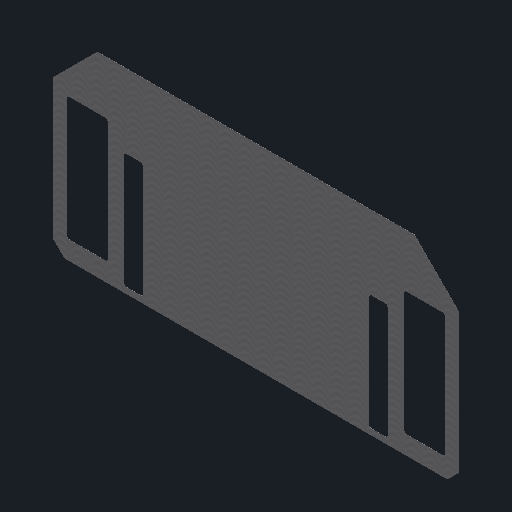
# Autodesk Inventor part: PlanchaBaseInferior
Saved by Autodesk Inventor 2022 (Build 260153000, 153)
## iProperties
Created: 2021-09-22
Part Number: PlanchaBaseInferior
Material: Steel, Mild, Welded
Document SubType Name: Sheet Metal
Designer: Andres
Density: 7.85 g/cm^3
Sheet Metal Rule: Default_mm
Appearance: Weld - Steel Mild
Author: Andres
Autodesk Inventor part; units mm, degrees
ref_plane "YZ Plane" through (0, 0, 0) normal (1, 0, 0) x (0, 1, 0)
ref_plane "XZ Plane" through (0, 0, 0) normal (0, 1, 0) x (-1, 0, 0)
ref_plane "XY Plane" through (0, 0, 0) normal (0, 0, 1) x (1, 0, 0)
sketch "Sketch1" plane through (0, 0, 0) normal (0, 0, 1) x (1, 0, 0)
  line L0 (893.3076, -345.9853) -> (750.9853, -345.9853)
  line L1 (-16.337, -345.9853) -> (-29.0147, -333.3076)
  line L2 (-29.0147, -333.3076) -> (-29.0147, -13.663)
  line L3 (-29.0147, -13.663) -> (63.663, 79.0147)
  line L4 (63.663, 79.0147) -> (125.9853, 79.0147)
  line L5 (750.9853, 79.0147) -> (813.3076, 79.0147)
  line L6 (570.9853, 79.0147) -> (725.9853, 79.0147)
  line L7 (150.9853, 79.0147) -> (305.9853, 79.0147)
  line L8 (330.9853, 79.0147) -> (545.9853, 79.0147)
  line L9 (813.3076, 79.0147) -> (905.9853, -13.663)
  line L10 (905.9853, -13.663) -> (905.9853, -333.3076)
  line L11 (905.9853, -333.3076) -> (893.3076, -345.9853)
  line L12 (125.9853, -345.9853) -> (-16.337, -345.9853)
  line L13 (903.663, -370.9853) -> (750.9853, -370.9853)
  line L14 (930.9853, -343.663) -> (903.663, -370.9853)
  line L15 (930.9853, -3.3076) -> (930.9853, -343.663)
  line L16 (823.663, 104.0147) -> (930.9853, -3.3076)
  line L17 (53.3076, 104.0147) -> (823.663, 104.0147)
  line L18 (-54.0147, -3.3076) -> (53.3076, 104.0147)
  line L19 (-54.0147, -343.663) -> (-54.0147, -3.3076)
  line L20 (-26.6924, -370.9853) -> (-54.0147, -343.663)
  line L21 (125.9853, -370.9853) -> (-26.6924, -370.9853)
  line L22 (750.9853, -370.9853) -> (125.9853, -370.9853)
  line L23 (125.9853, -370.9853) -> (125.9853, -345.9853)
  line L24 (125.9853, 79.0147) -> (125.9853, 91.5147)
  line L25 (125.9853, 91.5147) -> (150.9853, 91.5147)
  line L26 (150.9853, 79.0147) -> (150.9853, 91.5147)
  line L27 (305.9853, 91.5147) -> (305.9853, 79.0147)
  line L28 (305.9853, 91.5147) -> (330.9853, 91.5147)
  line L29 (330.9853, 91.5147) -> (330.9853, 79.0147)
  line L30 (545.9853, 91.5147) -> (545.9853, 79.0147)
  line L31 (545.9853, 91.5147) -> (570.9853, 91.5147)
  line L32 (570.9853, 91.5147) -> (570.9853, 79.0147)
  line L33 (725.9853, 79.0147) -> (725.9853, 91.5147)
  line L34 (725.9853, 91.5147) -> (750.9853, 91.5147)
  line L35 (750.9853, 79.0147) -> (750.9853, 91.5147)
  line L36 (750.9853, -370.9853) -> (750.9853, -345.9853)
extrude "Plate1" add sketch "Sketch1" along normal blind 0.5
sketch "Sketch2" plane through (0, 0, 0.5) normal (0, 0, 1) x (1, 0, 0)
  line L0 (78.4853, -25.4853) -> (-21.5147, -25.4853)
  line L1 (-21.5147, -25.4853) -> (-21.5147, -325.4853)
  line L2 (-21.5147, -325.4853) -> (78.4853, -325.4853)
  line L3 (78.4853, -325.4853) -> (78.4853, -25.4853)
  line L4 (78.4853, -25.4853) -> (-21.5147, -325.4853) construction
  line L5 (-21.5147, -25.4853) -> (78.4853, -325.4853) construction
  line L6 (119.5571, -370.4853) -> (-26.4853, -370.4853)
  line L7 (-26.4853, -370.4853) -> (-53.5147, -343.4558)
  line L8 (-53.5147, -343.4558) -> (-53.5147, -3.5147)
  line L9 (-53.5147, -3.5147) -> (53.5147, 103.5147)
  line L10 (53.5147, 103.5147) -> (823.4558, 103.5147)
  line L11 (823.4558, 103.5147) -> (930.4853, -3.5147)
  line L12 (930.4853, -3.5147) -> (930.4853, -343.4558)
  line L13 (930.4853, -343.4558) -> (903.4558, -370.4853)
  line L14 (903.4558, -370.4853) -> (757.4135, -370.4853)
  line L15 (893.5147, -346.4853) -> (757.4135, -346.4853)
  line L16 (906.4853, -333.5147) -> (893.5147, -346.4853)
  line L17 (906.4853, -13.4558) -> (906.4853, -333.5147)
  line L18 (813.5147, 79.5147) -> (906.4853, -13.4558)
  line L19 (757.4135, 79.5147) -> (813.5147, 79.5147)
  line L20 (577.4135, 79.5147) -> (719.5571, 79.5147)
  line L21 (337.4135, 79.5147) -> (539.5571, 79.5147)
  line L22 (63.4558, 79.5147) -> (119.5571, 79.5147)
  line L23 (157.4135, 79.5147) -> (299.5571, 79.5147)
  line L24 (-29.5147, -13.4558) -> (63.4558, 79.5147)
  line L25 (-29.5147, -333.5147) -> (-29.5147, -13.4558)
  line L26 (-16.5442, -346.4853) -> (-29.5147, -333.5147)
  line L27 (119.5571, -346.4853) -> (-16.5442, -346.4853)
  line L28 (438.4853, 188.8971) -> (438.4853, -449.5258) construction
  line L29 (798.4853, -25.4853) -> (898.4853, -25.4853)
  line L30 (898.4853, -25.4853) -> (898.4853, -325.4853)
  line L31 (898.4853, -325.4853) -> (798.4853, -325.4853)
  line L32 (798.4853, -325.4853) -> (798.4853, -25.4853)
  line L33 (798.4853, -25.4853) -> (898.4853, -325.4853) construction
  line L34 (898.4853, -25.4853) -> (798.4853, -325.4853) construction
  line L35 (119.5571, -346.4853) -> (119.5571, -370.4853)
  line L36 (757.4135, -370.4853) -> (757.4135, -346.4853)
  line L37 (757.4135, 79.5147) -> (757.4135, 91.5147)
  line L38 (757.4135, 91.5147) -> (719.5571, 91.5147)
  line L39 (719.5571, 91.5147) -> (719.5571, 79.5147)
  line L40 (577.4135, 79.5147) -> (577.4135, 91.5147)
  line L41 (577.4135, 91.5147) -> (539.5571, 91.5147)
  line L42 (539.5571, 91.5147) -> (539.5571, 79.5147)
  line L43 (337.4135, 79.5147) -> (337.4135, 91.5147)
  line L44 (337.4135, 91.5147) -> (299.5571, 91.5147)
  line L45 (299.5571, 91.5147) -> (299.5571, 79.5147)
  line L46 (157.4135, 79.5147) -> (157.4135, 91.5147)
  line L47 (157.4135, 91.5147) -> (119.5571, 91.5147)
  line L48 (119.5571, 91.5147) -> (119.5571, 79.5147)
  point P0 (0, 0)
  point P1 (28.4853, -175.4853)
  point P2 (438.4853, 79.5147)
  point P3 (848.4853, -175.4853)
  dimension "d1" = 100
  dimension "d2" = 300
  dimension "d4" = 410
  dimension "d5" = 255
  constraints: 96 end point, 5 midpoint, 5 symmetric about line, 2 parallel, 1 horizontal, 1 perpendicular, 1 vertical, 1 vertical alignment, 3 other
  measures "d1" distance between parallel lines of L1 L3
  measures "d2" distance between parallel lines of L2 L0
  measures "d4" distance from line of point (28.485, -175.485) L28
  measures "d5" vertical distance of point (438.485, 79.515) point (28.485, -175.485)
extrude "Cut1" cut sketch "Sketch2" against normal through all contours L3 L2 L1 L0 | L29 L30 L31 L32
fillet "Corner Round1" radius 6 8 edges at (78.4853, -25.4853, 0.25) (-21.5147, -25.4853, 0.25) (-21.5147, -325.4853, 0.25) (78.4853, -325.4853, 0.25) (898.4853, -25.4853, 0.25) (798.4853, -25.4853, 0.25) (898.4853, -325.4853, 0.25) (798.4853, -325.4853, 0.25)
sketch "Boceto3" plane through (0, 0, 0.5) normal (0, 0, 1) x (1, 0, 0)
  line L0 (123.4853, -355.9853) -> (158.4853, -355.9853)
  line L1 (163.4853, -350.9853) -> (163.4853, -80.9853)
  line L2 (158.4853, -75.9853) -> (123.4853, -75.9853)
  line L3 (118.4853, -80.9853) -> (118.4853, -350.9853)
  line L4 (78.4853, -31.4853) -> (78.4853, -319.4853) projected
  line L5 (438.4853, 103.5147) -> (438.4853, -370.4853)
  line L6 (753.4853, -355.9853) -> (718.4853, -355.9853)
  line L7 (713.4853, -350.9853) -> (713.4853, -80.9853)
  line L8 (718.4853, -75.9853) -> (753.4853, -75.9853)
  line L9 (758.4853, -80.9853) -> (758.4853, -350.9853)
  arc A0 (158.4853, -355.9853) -> (163.4853, -350.9853) centre (158.4853, -350.9853) ccw
  arc A1 (118.4853, -350.9853) -> (123.4853, -355.9853) centre (123.4853, -350.9853) ccw
  arc A2 (123.4853, -75.9853) -> (118.4853, -80.9853) centre (123.4853, -80.9853) ccw
  arc A3 (163.4853, -80.9853) -> (158.4853, -75.9853) centre (158.4853, -80.9853) ccw
  arc A4 (758.4853, -80.9853) -> (753.4853, -75.9853) centre (753.4853, -80.9853) ccw
  arc A5 (718.4853, -75.9853) -> (713.4853, -80.9853) centre (718.4853, -80.9853) ccw
  arc A6 (713.4853, -350.9853) -> (718.4853, -355.9853) centre (718.4853, -350.9853) ccw
  arc A7 (753.4853, -355.9853) -> (758.4853, -350.9853) centre (753.4853, -350.9853) ccw
  line L10 (903.663, -370.9853) -> (-26.6924, -370.9853) projected
  point P0 (0, 0)
  point P1 (118.4853, -355.9853)
  point P2 (163.4853, -355.9853)
  point P3 (163.4853, -75.9853)
  point P4 (118.4853, -75.9853)
  point P5 (758.4853, -355.9853)
  point P6 (713.4853, -355.9853)
  point P7 (713.4853, -75.9853)
  point P8 (758.4853, -75.9853)
  dimension "d9" = 45
  dimension "d10" = 280
  dimension "d13" = 5
  dimension "d16" = 275
  dimension "d17" = 15
  constraints: 18 end point, 16 point on circle, 16 point on line, 16 tangent, 8 centre point, 7 equal radius, 4 symmetric about line, 3 perpendicular, 1 horizontal
  measures "d9" distance of point (163.485, -75.985) point (118.485, -75.985)
  measures "d10" distance of point (163.485, -355.985) point (163.485, -75.985)
  measures "d13" radius of A0
  measures "d16" distance between parallel lines of L5 L1
  measures "d17" distance between parallel lines of L10 L0
extrude "Cortar2" cut sketch "Boceto3" against normal blind 0.5
equation "\"d6\" = Thickness"
equation "\"d14\" = Thickness"
equation "\"d0\" = Thickness"
equation "\"BendRadius\" = Thickness"
equation "\"BendReliefWidth\" = Thickness"
equation "\"BendReliefDepth\" = 0.5 * Thickness"
equation "\"CornerReliefSize\" = 4 * Thickness"
equation "\"MinimumRemnant\" = 2 * Thickness"
equation "\"TransitionRadius\" = BendRadius"
equation "\"JacobiRadiusSize\" = BendRadius"
equation "\"GapSize\" = Thickness"
equation "\"Thickness\" = 0.5"
body "Solid1"
